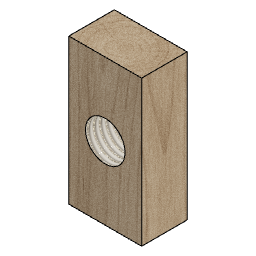
Moravian Workbench 2020 (Autodesk Fusion 360 archive; units mm, degrees)
design "Nut"
Autodesk Fusion 360 part; units mm, degrees
sketch "Sketch1" plane through (0, 0, 0) normal (0, 1, 0) x (1, 0, 0) in component "Nut_template"
  line L0 (0, 0) -> (101.6, 0)
  line L1 (101.6, 0) -> (101.6, -203.2)
  line L2 (101.6, -203.2) -> (0, -203.2)
  line L3 (0, -203.2) -> (0, 0)
  circle A0 centre (50.8, -101.6) radius 31.75
  line L4 (0, -203.2) -> (101.6, 0) construction
  line L5 (0, 0) -> (101.6, -203.2) construction
  point P0 (50.8, -101.6)
  dimension "d38" = 101.6
  dimension "d39" = 203.2
  dimension "d40" = 63.5
  constraint horizontal L0
  constraint vertical L1
  constraint horizontal L2
  constraint vertical L3
  constraint coincident L0.start L3.end
  constraint midpoint L5 P0
  constraint coincident P0 A0.centre
  measures "d38" distance of L1.end L2.end
  measures "d39" distance of L0.start L2.end
  measures "d40" diameter of A0
extrude "Extrude1" add sketch "Sketch1" along normal blind 63.5 in component "Nut_template"
thread "Thread1" "ACME Screw Threads 2 1/2 2.5000 4G" major diameter 64.262 minor diameter 55.2475 pitch 8.4667 angle 29 resizes the face on face at (82.5105, 42.3333, 103.1826) in component "Nut_template"
component "Nut_template" placed x (1, 0, 0) y (0, 1, 0) z (0, 0, 1) at (0, 0, 0)
equation "d38 = nut_width"
equation "d39 = nut_length"
equation "d40 = screw_diameter"
equation "d41 = nut_thickness"
equation "screw_diameter = 2.5 in"
equation "nut_thickness = 2.5 in"
equation "nut_length = 8 in"
equation "nut_width = 4 in"
equation "height_Ref = 34 in"
equation "length_Ref = 84 in"
equation "width_Ref = 24 in"
equation "cabinet_thickness_Ref = 0.75 in"
equation "chamfer_large_Ref = 0.5 in"
equation "chamfer_medium_Ref = 0.25 in"
equation "chamfer_small_Ref = 0.125 in"
equation "dogHole_length_Ref = 1 in"
equation "dogHole_setback_Ref = 1.75 in"
equation "dogHole_spacing_Ref = 4 in"
equation "dogHole_width_Ref = 0.75 in"
equation "dovetail_angle_Ref = 18 deg"
equation "leg_angle_Ref = 10 deg"
equation "leg_shoulderWidth_Ref = 0.25 in"
equation "leg_thickness_Ref = 4 in"
equation "leg_width_Ref = 5 in"
equation "panelGroove_width_Ref = 0.25 in"
equation "screw_diameter_Ref = 2.5 in"
equation "shoulder_width_Ref = 0.5 in"
equation "stretcher_thickness_Ref = 2 in"
equation "stretcher_width_Ref = 4 in"
equation "tenon_length_Ref = 1.5 in"
equation "top_leftOverhang_Ref = 6 in"
equation "top_rightOverhang_Ref = 20 in"
equation "top_thickness_Ref = 4 in"
equation "wagonVise_topThickness_Ref = 1 in"
equation "dog_headHeight_Ref = 1 in"
equation "lvScrew_height_Ref = 22 in"
equation "lvGuide_width_Ref = 3 in"
equation "lvGuide_thickness_Ref = 1 in"
equation "lvGuide_height_Ref = 6 in"
equation "nut_thickness_Ref = 2 in"
equation "nut_length_Ref = 8 in"
equation "nut_width_Ref = 4 in"
equation "garter_thickness_Ref = 0.25 in"
equation "handle_diameter_Ref = 1 in"
equation "garter_width_Ref = 4 in"
equation "lvPin_diameter_Ref = 0.5 in"
equation "endCap_thickness_Ref = 2.5 in"
equation "screw_length_Ref = 24 in"
equation "screw_hubLength_Ref = 4 in"
